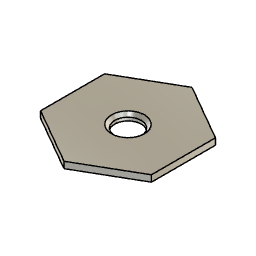
Core_PartB_x1 (Autodesk Fusion 360 design; units mm, degrees)
Autodesk Fusion 360 part; units mm, degrees
sketch "Sketch1" plane through (0, 0, 0) normal (0, 0, 1) x (1, 0, 0)
  line L0 (13, 7.5056) -> (0, 15.0111)
  line L1 (0, 15.0111) -> (-13, 7.5056)
  line L2 (-13, 7.5056) -> (-13, -7.5056)
  line L3 (-13, -7.5056) -> (0, -15.0111)
  line L4 (0, -15.0111) -> (13, -7.5056)
  line L5 (13, -7.5056) -> (13, 7.5056)
  dimension "d1" = 13
  measures "d1" distance of origin L5
extrude "Extrude1" add sketch "Sketch1" along normal blind 1.5
sketch "Sketch2" plane through (0, 0, 1.5) normal (0, 0, 1) x (-1, 0, 0)
  line L0 (-13, 7.5056) -> (-13, -7.5056)
  line L1 (-13, -7.5056) -> (0, -15.0111)
  line L2 (0, -15.0111) -> (13, -7.5056)
  line L3 (13, -7.5056) -> (13, 7.5056)
  line L4 (13, 7.5056) -> (0, 15.0111)
  line L5 (0, 15.0111) -> (-13, 7.5056)
  circle A0 centre (0, 0) radius 3.1
  dimension "d4" = 6.2
  constraint coincident A0.centre origin
  measures "d4" diameter of A0
extrude "Extrude2" cut sketch "Sketch2" against normal blind 13 contours A0
chamfer "Chamfer1" distance 0.75 angle 45 1 edges at (2.8902, -1.121, 1.5)
